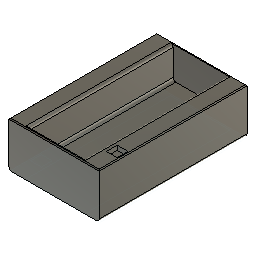
pinecil case (Autodesk Fusion 360 design; units mm, degrees)
Autodesk Fusion 360 part; units mm, degrees
sketch "Sketch1" plane through (0, 0, 0) normal (0, 1, 0) x (1, 0, 0)
  line L0 (0, 0) -> (0, -47)
  line L1 (3, -50) -> (20, -50)
  line L2 (20, -32) -> (20, -3)
  line L3 (17, 0) -> (0, 0)
  line L4 (20, -50) -> (97, -50)
  line L5 (100, -47) -> (100, -35)
  line L6 (77, -35) -> (23, -35)
  line L7 (100, -35) -> (80, -35)
  line L8 (80, -32) -> (80, -3)
  line L9 (83, 0) -> (100, 0)
  line L10 (100, 0) -> (100, -35)
  arc A0 (0, -47) -> (3, -50) centre (3, -47) ccw
  arc A1 (97, -50) -> (100, -47) centre (97, -47) ccw
  arc A2 (83, 0) -> (80, -3) centre (83, -3) ccw
  arc A3 (20, -3) -> (17, 0) centre (17, -3) ccw
  arc A4 (20, -32) -> (23, -35) centre (23, -32) ccw
  arc A5 (77, -35) -> (80, -32) centre (77, -32) ccw
  dimension "d1" = 3
  constraint coincident L0.start L3.end
  constraint vertical L0
  constraint perpendicular L0 L1
  constraint perpendicular L1 L2
  constraint perpendicular L0 L3
  constraint perpendicular L2 L4
  constraint perpendicular L1 L5
  constraint perpendicular L2 L6
  constraint coincident L6 L7.end
  constraint perpendicular L6 L8
  constraint perpendicular L8 L9
  constraint perpendicular L6 L10
  constraint tangent L1 A0
  constraint tangent L0 A0
  constraint tangent L5 A1
  constraint tangent L4 A1
  constraint equal A0 A1
  constraint tangent L8 A2
  constraint tangent L9 A2
  constraint equal A0 A2
  constraint tangent L2 A3
  constraint tangent L3 A3
  constraint equal A0 A3
  constraint coincident L1.end L2
  constraint tangent L6 A4
  constraint tangent L2 A4
  constraint equal A0 A4
  constraint coincident L7.end L8
  constraint coincident L5.end L6
  constraint tangent L8 A5
  constraint tangent L6 A5
  constraint equal A0 A5
  measures "d1" radius of A0
extrude "Extrude1" add sketch "Sketch1" against normal blind 10 makes body 1
sketch "Sketch2" plane through (0, -10, 0) normal (0, -1, 0) x (1, 0, 0)
  line L0 (20, 3) -> (20, 32)
  arc A0 (23, 35) -> (20, 32) centre (23, 32) ccw
  line L1 (23, 35) -> (77, 35)
  arc A1 (80, 32) -> (77, 35) centre (77, 32) ccw
  line L2 (80, 32) -> (80, 3)
  arc A2 (80, 3) -> (83, 0) centre (83, 3) ccw
  line L3 (83, 0) -> (100, 0)
  line L4 (100, 0) -> (100, 47)
  arc A3 (100, 47) -> (97, 50) centre (97, 47) ccw
  line L5 (97, 50) -> (3, 50)
  arc A4 (3, 50) -> (0, 47) centre (3, 47) ccw
  line L6 (0, 47) -> (0, 0)
  line L7 (0, 0) -> (17, 0)
  arc A5 (17, 0) -> (20, 3) centre (17, 3) ccw
extrude "Extrude2" add sketch "Sketch2" along normal blind 150 bodies 1
sketch "Sketch3" plane through (0, -160, 0) normal (0, -1, 0) x (1, 0, 0)
  line L0 (80, 32) -> (80, 3)
  arc A0 (80, 3) -> (83, 0) centre (83, 3) ccw
  line L1 (83, 0) -> (100, 0)
  line L2 (100, 0) -> (100, 47)
  arc A1 (100, 47) -> (97, 50) centre (97, 47) ccw
  line L3 (97, 50) -> (3, 50)
  arc A2 (3, 50) -> (0, 47) centre (3, 47) ccw
  line L4 (0, 47) -> (0, 0)
  line L5 (0, 0) -> (17, 0)
  arc A3 (17, 0) -> (20, 3) centre (17, 3) ccw
  line L6 (20, 3) -> (20, 32)
  arc A4 (23, 35) -> (20, 32) centre (23, 32) ccw
  line L7 (23, 35) -> (77, 35)
  arc A5 (80, 32) -> (77, 35) centre (77, 32) ccw
  line L8 (100, 0) -> (0, 0)
  line L9 (0, 0) -> (0, 45)
  line L10 (0, 45) -> (100, 45)
  line L11 (100, 45) -> (100, 0)
  constraint horizontal L8
  constraint vertical L9
  constraint horizontal L10
  constraint vertical L11
  constraint coincident L4 L9.end
  constraint coincident L1.end L2.start
extrude "Extrude3" add sketch "Sketch3" along normal blind 2 bodies 1
sketch "Sketch4" plane through (0, 0, 0) normal (0, 1, 0) x (-1, 0, 0)
  line L0 (-20, 32) -> (-20, 3)
  arc A0 (-20, 3) -> (-17, 0) centre (-17, 3) ccw
  line L1 (-17, 0) -> (0, 0)
  line L2 (0, 0) -> (0, 47)
  arc A1 (0, 47) -> (-3, 50) centre (-3, 47) ccw
  line L3 (-3, 50) -> (-97, 50)
  arc A2 (-97, 50) -> (-100, 47) centre (-97, 47) ccw
  line L4 (-100, 47) -> (-100, 0)
  line L5 (-100, 0) -> (-83, 0)
  arc A3 (-83, 0) -> (-80, 3) centre (-83, 3) ccw
  line L6 (-80, 3) -> (-80, 32)
  arc A4 (-77, 35) -> (-80, 32) centre (-77, 32) ccw
  line L7 (-77, 35) -> (-23, 35)
  arc A5 (-20, 32) -> (-23, 35) centre (-23, 32) ccw
  line L8 (0, 0) -> (-100, 0)
  line L9 (-100, 0) -> (-100, 40)
  line L10 (-100, 40) -> (0, 40)
  line L11 (0, 40) -> (0, 0)
  constraint horizontal L8
  constraint vertical L9
  constraint horizontal L10
  constraint vertical L11
  constraint coincident L1.end L2.start
extrude "Extrude4" add sketch "Sketch4" along normal blind 2 bodies 1
sketch "Sketch5" plane through (0, 0, 0) normal (0, 0, -1) x (1, 0, 0)
  line L0 (17, 0) -> (17, 160)
  line L1 (17, 160) -> (83, 160)
  line L2 (83, 160) -> (83, 0)
  line L3 (83, 0) -> (17, 0)
  line L4 (0, 162) -> (0, -2)
  line L5 (0, -2) -> (100, -2)
  line L6 (100, -2) -> (100, 162)
  line L7 (100, 162) -> (0, 162)
extrude "Extrude5" add sketch "Sketch5" 1 faces at (5.6667, -106.6667, 0) along normal blind 2 separate body contours L0 L1 L2 L3 on bodies 1 makes body 2
move_body "Move1" bodies 2 to x (1, 0, 0) y (0, 1, 0) z (0, 0, 1) at (0, 0, -5)
sketch "Sketch6" plane through (0, 0, 0) normal (0, 0, -1) x (1, 0, 0)
  line L0 (17, 0) -> (17, 160)
  line L1 (17, 160) -> (83, 160)
  line L2 (83, 160) -> (83, 0)
  line L3 (83, 0) -> (17, 0)
  line L4 (0, 162) -> (0, -2)
  line L5 (0, -2) -> (100, -2)
  line L6 (100, -2) -> (100, 162)
  line L7 (100, 162) -> (0, 162)
  line L8 (14, 140) -> (2, 140)
  line L9 (2, 140) -> (2, 128)
  line L10 (2, 128) -> (14, 128)
  line L11 (14, 128) -> (14, 140)
  constraint horizontal L8
  constraint vertical L9
  constraint horizontal L10
  constraint vertical L11
extrude "Extrude6" cut sketch "Sketch6" against normal blind 5 contours L8 L9 L10 L11 bodies 1
sketch "Sketch7" plane through (0, 0, 0) normal (0, 0, -1) x (1, 0, 0)
  line L0 (2, 140) -> (14, 140)
  line L1 (14, 140) -> (14, 128)
  line L2 (14, 128) -> (2, 128)
  line L3 (2, 128) -> (2, 140)
  line L4 (17, 0) -> (17, 160)
  line L5 (17, 160) -> (83, 160)
  line L6 (83, 160) -> (83, 0)
  line L7 (83, 0) -> (17, 0)
  line L8 (0, 162) -> (0, -2)
  line L9 (0, -2) -> (100, -2)
  line L10 (100, -2) -> (100, 162)
  line L11 (100, 162) -> (0, 162)
chamfer "Chamfer1" distance 1 angle 45 4 edges at (100, -80, 0) (50, 2, 0) (0, -80, 0) (50, -162, 0) on bodies 1
move_body "Move2" bodies 1 to x (-1, 0, 0) y (0, 1, 0) z (0, 0, -1) at (100, 0, 51)
hidden bodies 2
